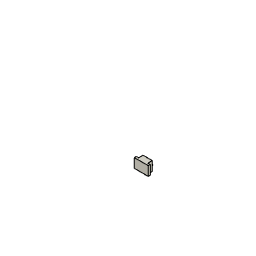
Taste_rechts (Autodesk Fusion 360 design; units mm, degrees)
Autodesk Fusion 360 part; units mm, degrees
sketch "Skizze1" plane through (0, 0, 59.536) normal (0, 0, -1) x (1, 0, 0)
  line L0 (54.288, -85.97) -> (62.288, -85.97)
  line L1 (62.288, -85.97) -> (62.288, -82.97)
  line L2 (62.288, -82.97) -> (54.288, -82.97)
  line L3 (54.288, -82.97) -> (54.288, -85.97)
  line L4 (64.188, -82.82) -> (62.188, -82.82)
  line L5 (62.188, -82.82) -> (62.188, -86.47)
  line L6 (62.188, -86.47) -> (54.388, -86.47)
  line L7 (54.388, -86.47) -> (54.388, -82.82)
  line L8 (54.388, -82.82) -> (52.388, -82.82)
  line L9 (52.388, -82.82) -> (52.388, -81.07)
  line L10 (52.388, -81.07) -> (64.188, -81.07)
  line L11 (64.188, -81.07) -> (64.188, -82.82)
  line L12 (50.288, -82.97) -> (50.288, -85.97)
  line L13 (40.65, -82.97) -> (67.1, -82.97)
  line L14 (-54.35, -82.97) -> (27.15, -82.97)
  line L15 (56.538, -80.97) -> (60.038, -80.97)
  point P0 (54.288, -85.97)
  point P1 (50.288, -85.97)
  dimension "d132_1_2_4_1" = 0.1
  dimension "d133_1_2_4_1" = 0.1
  dimension "d137_1_2_4_1" = 0.5
  dimension "d139_1_2_4_1" = 2
  dimension "d140_1_2_4_1" = 2
  dimension "d498" = 0.15
  dimension "d499" = 0.1
  constraint horizontal L4
  constraint perpendicular L0 L5
  constraint perpendicular L5 L6
  constraint perpendicular L0 L7
  constraint perpendicular L7 L8
  constraint perpendicular L0 L9
  constraint perpendicular L7 L10
  constraint perpendicular L10 L11
  constraint horizontal L4.end L7.end
  measures "d132_1_2_4_1" distance of L1 L5
  measures "d133_1_2_4_1" distance of L3 L7
  measures "d137_1_2_4_1" distance of L0 L6
  measures "d139_1_2_4_1" distance of L7.end L8.end
  measures "d140_1_2_4_1" distance of L4.start L4.end
  measures "d498" distance of L4 L13
  measures "d499" distance of L10 L15
extrude "Extrusion1" add sketch "Skizze1" along normal blind 7.8 contours L0 L2 L5 L7 L13 | L0 L5 L6 L7 | L2 L4 L5 L7 L8 L9 L10 L11 L13
sketch "Skizze2" plane through (0, 86.47, 0) normal (0, 1, 0) x (-1, 0, 0)
  line L0 (-62.188, 59.536) -> (-62.188, 51.736)
  line L1 (-62.188, 51.736) -> (-54.388, 51.736)
  line L2 (-54.388, 51.736) -> (-54.388, 59.536)
  line L3 (-1.1828, 57.6693) -> (-1.1828, 54.5)
  line L4 (-1.1828, 54.5) -> (1.7303, 54.5)
  line L5 (1.7303, 54.5) -> (1.7303, 53.1394)
  line L6 (1.7303, 53.1394) -> (4.964, 56.0847)
  line L7 (4.964, 56.0847) -> (2.7592, 58.2974)
  line L8 (2.7592, 58.2974) -> (2.7592, 57)
  line L9 (2.7592, 57) -> (-1, 57)
  line L10 (-61.488, 56.386) -> (-61.488, 54.886)
  line L11 (-61.488, 54.886) -> (-58.488, 54.886)
  line L12 (-58.488, 54.886) -> (-58.488, 53.236)
  line L13 (-58.488, 53.236) -> (-55.088, 55.636)
  line L14 (-55.088, 55.636) -> (-58.488, 58.036)
  line L15 (-58.488, 58.036) -> (-58.488, 56.386)
  line L16 (-58.488, 56.386) -> (-61.488, 56.386)
  line L17 (-62.188, 59.536) -> (-54.388, 59.536)
  point P0 (-62.188, 55.636)
  point P1 (-61.488, 55.636)
  dimension "d391" = 1.5
  dimension "d392" = 1.5
  dimension "d393" = 1.5
  dimension "d394" = 0.7
  dimension "d395" = 3
  dimension "d396" = 0.7
  constraint vertical L3
  constraint perpendicular L3 L4
  constraint perpendicular L4 L5
  constraint parallel L5 L8
  constraint perpendicular L8 L9
  constraint vertical L10
  constraint perpendicular L10 L11
  constraint perpendicular L11 L12
  constraint parallel L12 L15
  constraint horizontal L16
  constraint midpoint L0 P0
  constraint midpoint L10 P1
  constraint horizontal P0 P1
  constraint horizontal L13.end P0
  constraint vertical L11.end L15.end
  measures "d391" distance of L10.start L10.end
  measures "d392" distance of L14.end L17
  measures "d393" distance of L1 L12.end
  measures "d394" distance of L2 L13.end
  measures "d395" distance of L10.start L15.end
  measures "d396" distance of L0 L10
emboss "Prägen1" depth 1 profiles "Skizze2" section 1 contours L10 L11 L12 L13 L14 L15 L16 onto face at (59.588, 86.47, 54.336)
move_body "Verschieben2" bodies 1 to x (1, 0, 0) y (0, 1, 0) z (0, 0, 1) at (12, 0, -35.8)
equation "d133_1_2_4_1 = d132_1_2_4_1"
equation "d139_1_2_4_1 = 4.00 mm / 2"
equation "d140_1_2_4_1 = d139_1_2_4_1"
equation "d393 = d392"
